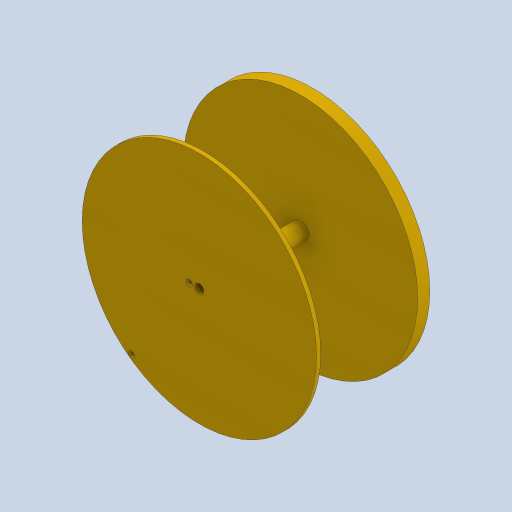
# Autodesk Inventor part: Bobbin_x_b
Saved by Autodesk Inventor 2024 (Build 280153000, 153)
## iProperties
Created: 2022-01-24
Part Number: Bobbin_x_b
Material: Generic
Document SubType Name: Modeling
Designer: frede
Density: 1 g/cm^3
Appearance: Default
Author: frede
Autodesk Inventor part; units mm, degrees
ref_plane "YZ Plane" through (0, 0, 0) normal (1, 0, 0) x (0, 1, 0)
ref_plane "XZ Plane" through (0, 0, 0) normal (0, 1, 0) x (-1, 0, 0)
ref_plane "XY Plane" through (0, 0, 0) normal (0, 0, 1) x (1, 0, 0)
sketch "Sketch1" plane through (0, 0, 0) normal (0, 0, 1) x (1, 0, 0)
  circle A0 centre (0, 0) radius 29
  dimension "d0" = 58
  constraints: 1 centre point, 1 coincident
  measures "d0" diameter of A0
extrude "Extrusion1" add sketch "Sketch1" along normal blind 3
sketch "Sketch2" plane through (0, 0, 3) normal (0, 0, 1) x (1, 0, 0)
  circle A0 centre (0, 0) radius 2
  dimension "d3" = 4
  constraints: 1 centre point, 1 coincident
  measures "d3" diameter of A0
extrude "Extrusion2" add sketch "Sketch2" along normal blind 24
sketch "Sketch3" plane through (0, 0, 27) normal (0, 0, 1) x (1, 0, 0)
  circle A0 centre (0, 0) radius 29
  dimension "d6" = 58
  constraints: 1 centre point, 1 coincident
  measures "d6" diameter of A0
extrude "Extrusion3" add sketch "Sketch3" along normal blind 1
sketch "Sketch4" plane through (0, 0, 28) normal (0, 0, 1) x (1, 0, 0)
  circle A0 centre (0, 0) radius 1.1
  dimension "d9" = 2.2
  constraints: 1 centre point, 1 coincident
  measures "d9" diameter of A0
extrude "Extrusion4" cut sketch "Sketch4" against normal through all
sketch "Sketch6" plane through (0, 0, 28) normal (0, 0, 1) x (1, 0, 0)
  circle A0 centre (0, 0) radius 2 construction
  circle A1 centre (-16.8114, -22.5) radius 0.4
  circle A2 centre (-2.5, 0) radius 0.4
  circle A3 centre (0, 0) radius 29 projected
  dimension "d20" = 0.8
  dimension "d21" = 0.8
  dimension "d32" = 2.5
  dimension "d41" = 22.5
  constraints: 2 centre point
  measures "d20" diameter of A1
  measures "d21" diameter of A2
  measures "d32" distance of A2.centre point (0, 0)
  measures "d41" vertical distance of A3.centre A1.centre
sketch "Sketch7" plane through (0, 0, 28) normal (0, 0, 1) x (1, 0, 0)
  point P0 (0, 0)
extrude "Extrusion5" cut sketch "Sketch6" against normal up to surface (1 mm away) contours A1 | A2
chamfer "Chamfer1" distance 0.4 angle 45 2 edges at (-2.9, 0, 28) (-17.2114, -22.5, 28)
sketch "Sketch9" plane through (0, 0, 0) normal (0, 0, -1) x (-1, 0, 0)
  point P0 (0, 0)
  point P1 (11, -11.5)
  point P2 (-11, -11.5)
  point P3 (11, -16.5)
  point P4 (-11, -16.5)
  dimension "d44" = 11
  dimension "d45" = 11
  dimension "d46" = 11.5
  dimension "d47" = 11.5
  dimension "d48" = 5
  dimension "d49" = 5
  measures "d44" horizontal distance of point (0, 0) point (11, -11.5)
  measures "d45" horizontal distance of point (0, 0) point (-11, -11.5)
  measures "d46" vertical distance of point (0, 0) point (-11, -11.5)
  measures "d47" vertical distance of point (0, 0) point (11, -11.5)
  measures "d48" distance of point (11, -11.5) point (11, -16.5)
  measures "d49" distance of point (-11, -11.5) point (-11, -16.5)
hole "Hole2" at (11, -11.5, 0) at (-11, -11.5, 0) at (-11, -16.5, 0) at (11, -16.5, 0) direction (0, 0, 1) diameter 2.459 depth 2.8 thread size "M3x0.5" class "6H" standard "ISO Metric profile"
loft "Loft1" [suppressed]
body "Solid1"
body "Solid2"
